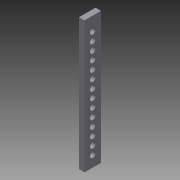
# Autodesk Inventor part: Handle-Cart Link
Saved by Autodesk Inventor 2014 (Build 180170000, 170)
## iProperties
Created: 2014-02-04
Part Number: Handle-Cart Link
Material: Generic
Document SubType Name: Modeling
Designer: Nitesh
Density: 1 g/cm^3
Appearance: Default
Author: Nitesh
Autodesk Inventor part; units mm, degrees
ref_plane "YZ Plane" through (0, 0, 0) normal (1, 0, 0) x (0, 1, 0)
ref_plane "XZ Plane" through (0, 0, 0) normal (0, 1, 0) x (-1, 0, 0)
ref_plane "XY Plane" through (0, 0, 0) normal (0, 0, 1) x (1, 0, 0)
sketch "Sketch1" plane through (0, 0, 0) normal (1, 0, 0) x (0, 1, 0)
  line L0 (0, 0) -> (152.4, 0)
  line L1 (152.4, 0) -> (152.4, 19.05)
  line L2 (152.4, 19.05) -> (0, 19.05)
  line L3 (0, 19.05) -> (0, 0)
  circle A0 centre (12.7, 9.525) radius 3.175
  circle A1 centre (22.225, 9.525) radius 3.175
  circle A2 centre (31.75, 9.525) radius 3.175
  circle A3 centre (41.275, 9.525) radius 3.175
  circle A4 centre (50.8, 9.525) radius 3.175
  circle A5 centre (60.325, 9.525) radius 3.175
  circle A6 centre (69.85, 9.525) radius 3.175
  circle A7 centre (79.375, 9.525) radius 3.175
  circle A8 centre (88.9, 9.525) radius 3.175
  circle A9 centre (98.425, 9.525) radius 3.175
  circle A10 centre (107.95, 9.525) radius 3.175
  circle A11 centre (117.475, 9.525) radius 3.175
  circle A12 centre (127, 9.525) radius 3.175
  circle A13 centre (136.525, 9.525) radius 3.175
  dimension "d0" = 19.05
  dimension "d1" = 152.4
  dimension "d2" = 6.35
  dimension "d3" = 12.7
  dimension "d4" = 9.525
  dimension "d7" = 9.525
  constraints: 14 centre point, 8 end point, 2 horizontal, 2 parallel, 1 perpendicular, 26 other
  measures "d0" distance of L2.end L0.start
  measures "d1" distance of L0.start L0.end
  measures "d2" diameter of A0
  measures "d3" distance from line of L3 A0.centre
  measures "d4" distance from line of L0 A0.centre
  measures "d7" distance of A0.centre A1.centre
extrude "Extrusion1" add sketch "Sketch1" along normal blind 6.35
body "Solid1"
